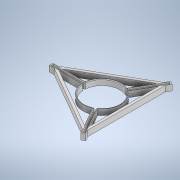
# Autodesk Inventor part: Konstruct
Saved by Autodesk Inventor 2020 (Build 240168000, 168)
## iProperties
Created: 2022-05-21
Part Number: Konstruct
Material: Generisch
Document SubType Name: Modeling
Designer: sp
Density: 1 g/cm^3
Appearance: Vorgabe
Author: sp
## iProperties of the stored document _3D-Druck.ipt
Created: 2022-05-21
Part Number: _3D-Druck
Material: Generisch
Document SubType Name: Modeling
Designer: sp
Density: 1 g/cm^3
Appearance: Vorgabe
Author: sp
Autodesk Inventor part; units mm, degrees
ref_plane "YZ Plane" through (0, 0, 0) normal (1, 0, 0) x (0, 1, 0)
ref_plane "XZ Plane" through (0, 0, 0) normal (0, 1, 0) x (-1, 0, 0)
ref_plane "XY Plane" through (0, 0, 0) normal (0, 0, 1) x (1, 0, 0)
sketch "Skizze1" plane through (0, 0, 0) normal (0, 1, 0) x (-1, 0, 0)
  circle A0 centre (0, 0) radius 31.25
  circle A1 centre (0, 0) radius 33
  line L0 (0, 109.2005) -> (0, -98.3382) construction
  line L1 (65.6021, 0) -> (-69.7309, 0) construction
  line L2 (-37.5074, 64.9647) -> (55.9703, -96.9435) construction
  line L3 (-38.0847, -65.9646) -> (43.9559, 76.1338) construction
  line L4 (30, 1.25) -> (87, 1.25)
  line L5 (87, 1.25) -> (87, -1.25)
  line L6 (87, -1.25) -> (30, -1.25)
  line L7 (30, -1.25) -> (30, 1.25)
  line L8 (28, -3.25) -> (89, -3.25)
  line L9 (89, -3.25) -> (89, 3.25)
  line L10 (89, 3.25) -> (28, 3.25)
  line L11 (28, 3.25) -> (28, -3.25)
  line L12 (-16.0825, 25.3558) -> (-44.5825, 74.7192)
  line L13 (-42.4175, 75.9692) -> (-13.9175, 26.6058)
  line L14 (-11.1854, 25.8737) -> (-41.6854, 78.7013)
  line L15 (-47.3146, 75.4513) -> (-16.8146, 22.6237)
  line L16 (-44.5825, 74.7192) -> (-42.4175, 75.9692)
  line L17 (-41.6854, 78.7013) -> (-47.3146, 75.4513)
  line L18 (-13.9175, 26.6058) -> (-16.0825, 25.3558)
  line L19 (-16.8146, 22.6237) -> (-11.1854, 25.8737)
  line L20 (-13.9175, -26.6058) -> (-42.4175, -75.9692)
  line L21 (-44.5825, -74.7192) -> (-16.0825, -25.3558)
  line L22 (-16.8146, -22.6237) -> (-47.3146, -75.4513)
  line L23 (-41.6854, -78.7013) -> (-11.1854, -25.8737)
  line L24 (-42.4175, -75.9692) -> (-44.5825, -74.7192)
  line L25 (-47.3146, -75.4513) -> (-41.6854, -78.7013)
  line L26 (-16.0825, -25.3558) -> (-13.9175, -26.6058)
  line L27 (-11.1854, -25.8737) -> (-16.8146, -22.6237)
  point P0 (-32.8011, 56.8131)
  point P1 (-32.8011, -56.8131)
  point P2 (32.8396, -3.25)
  point P3 (32.8396, 3.25)
  point P4 (-13.6052, 30.0649)
  point P5 (-19.2344, 26.8149)
  point P6 (-19.2344, -26.8149)
  point P7 (-13.6052, -30.0649)
  point P8 (31.225, -1.25)
  point P9 (-14.53, -27.6666)
  point P10 (-16.695, -26.4166)
  point P11 (-16.695, 26.4166)
  point P12 (-14.53, 27.6666)
  point P13 (31.225, 1.25)
  dimension "d0" = 62.5
  dimension "d1" = 66
  dimension "d2" = 120
  dimension "d3" = 120
  dimension "d4" = 2.5
  dimension "d5" = 2
  dimension "d6" = 57
  dimension "d7" = 30
  dimension "d10" = 360
  constraints: 56 end point, 6 perpendicular, 4 point on line, 2 centre point, 2 coincident, 1 horizontal, 1 parallel, 1 vertical, 56 other
  measures "d0" diameter of A0
  measures "d1" diameter of A1
  measures "d2" angle of L1 L2
  measures "d3" angle of L1 L3
  measures "d4" distance between parallel lines of L6 L4
  measures "d5" distance between parallel lines of L6 L8
  measures "d6" distance of L5.end L6.end
  measures "d7" distance from line of L7 point (0, 0)
extrude "Extrusion1" add sketch "Skizze1" along normal blind 10 contours A0 L10 A1 L4 | L6 A1 L8 A0 | A0 L14 A1 L10 | A1 L10 L9 L8 L6 L5 L4 | L8 A1 L23 A0 | A0 L13 A1 L14 | L23 A1 L20 A0 | A1 L13 L16 L12 L15 L17 L14 | L23 L25 L22 A1 L21 L24 L20 | A0 L15 A1 L12 | L21 A1 L22 A0 | A0 L22 A1 L15
fillet "Rundung1" radius 2 6 edges at (-31.225, 5, -1.25) (-31.225, 5, 1.25) (14.53, 5, 27.6666) (16.695, 5, 26.4166) (16.695, 5, -26.4166) (14.53, 5, -27.6666)
chamfer "Fase1" distance 1 angle 45 15 edges at (-15.625, 10, -27.0633) (14.3424, 10, -28.3783) (28.9402, 10, -52.6258) (-31.7475, 10, -1.7683) (-60.0454, 10, -1.25) (31.25, 10, 0) (17.4051, 10, 26.61) (31.1052, 10, 51.3758) (17.4051, 10, -26.61) (31.1052, 10, -51.3758) (-15.625, 10, 27.0633) (-31.7475, 10, 1.7683) (-60.0454, 10, 1.25) (14.3424, 10, 28.3783) (28.9402, 10, 52.6258)
sketch "Skizze2" plane through (0, 0, 0) normal (0, 1, 0) x (-1, 0, 0)
  line L0 (-47.3146, 75.4513) -> (-19.2344, 26.8149) projected
  line L1 (-38.5127, 60.2059) -> (-38.5127, -59.496)
  line L2 (-38.5127, -59.496) -> (-38.5127, -60.2059)
  line L3 (-19.2344, -26.8149) -> (-47.3146, -75.4513) projected
  line L4 (-42.8652, 67.7448) -> (-42.8652, -67.7448)
  line L5 (-42.8652, -59.496) -> (-42.8652, -60.2059)
  line L6 (-38.5127, 60.2059) -> (-42.8652, 67.7448)
  line L7 (-38.4567, -60.109) -> (-42.8652, -67.7448)
  line L8 (-32.8835, -63.4559) -> (70.7814, -3.605)
  line L9 (70.7814, -3.605) -> (71.3962, -3.25)
  line L10 (-37.2361, -70.9948) -> (80.1013, -3.25)
  line L11 (72.9577, -7.3744) -> (73.5725, -7.0194)
  line L12 (-32.8835, -63.4559) -> (-37.2361, -70.9948)
  line L13 (71.2843, -3.25) -> (80.1013, -3.25)
  line L14 (71.3962, 3.25) -> (-32.2687, 63.101)
  line L15 (-32.2687, 63.101) -> (-32.8835, 63.4559)
  line L16 (80.1013, 3.25) -> (-37.2361, 70.9948)
  line L17 (-30.0925, 66.8704) -> (-30.7073, 67.2254)
  line L18 (71.3962, 3.25) -> (80.1013, 3.25)
  line L19 (-32.8276, 63.359) -> (-37.2361, 70.9948)
  point P0 (0, 0)
  point P1 (-41.6854, -78.7013)
  point P2 (-13.6052, -30.0649)
  point P3 (32.8396, -3.25)
  point P4 (89, -3.25)
  point P5 (89, 3.25)
  point P6 (32.8396, 3.25)
  point P7 (-13.6052, 30.0649)
  point P8 (-41.6854, 78.7013)
  dimension "d20" = 360
  constraints: 36 end point, 11 point on line, 2 collinear, 1 vertical, 55 other
extrude "Extrusion2" add sketch "Skizze2" along normal blind 10
